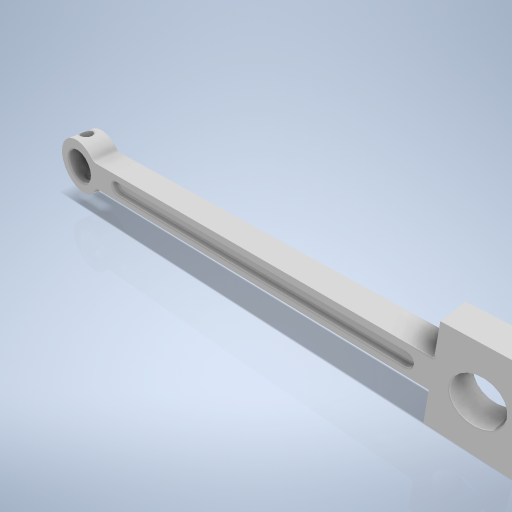
# Autodesk Inventor part: pleuel_rad_2
Saved by Autodesk Inventor 2024.2 (Build 282272000, 272)
## iProperties
Created: 2024-05-05
Part Number: pleuel_rad_2
Material: Generisch
Document SubType Name: Modeling
Designer: Fabri
Density: 1 g/cm^3
Appearance: Vorgabe
Author: Fabri
Autodesk Inventor part; units mm, degrees
ref_plane "YZ Plane" through (0, 0, 0) normal (1, 0, 0) x (0, 1, 0)
sketch "Skizze1" plane through (0, 0, 0) normal (0, 1, 0) x (-1, 0, 0)
  line L0 (0, 19.5) -> (-30, 19.5)
  line L1 (-30, 19.5) -> (-30, -19.5)
  line L2 (-30, -19.5) -> (0, -19.5)
  line L3 (0, -19.5) -> (0, 19.5)
  line L4 (0, 6) -> (169.4, 6)
  line L5 (169.4, 6) -> (169.4, -6)
  line L6 (169.4, -6) -> (0, -6)
  line L7 (0, -6) -> (0, 6)
  line L8 (0, 0) -> (-64.3399, 0) construction
  line L9 (9, 0) -> (145, 0) construction
  line L10 (9, 3) -> (145, 3)
  line L11 (145, -3) -> (9, -3)
  arc A0 (9, 3) -> (9, -3) centre (9, 0) ccw
  arc A1 (145, -3) -> (145, 3) centre (145, 0) ccw
  point P0 (169.4, 0)
  point P1 (-15, -19.5)
  point P2 (77, 0)
  point P3 (6, 0)
  point P4 (148, 0)
  dimension "d0" = 39
  dimension "d1" = 30
  dimension "d2" = 184.4
  dimension "d3" = 12
  dimension "d4" = 6
  dimension "d5" = 6
  dimension "d6" = 3
  dimension "d27" = 142
  constraints: 26 end point, 6 parallel, 6 point on circle, 4 midpoint, 4 tangent, 3 horizontal, 2 centre point, 2 perpendicular, 1 point on line, 1 symmetric about line, 2 other
  measures "d0" distance between parallel lines of L2 L0
  measures "d1" distance between parallel lines of L1 L3
  measures "d2" horizontal distance of point (-15, -19.5) point (169.4, 0)
  measures "d3" distance between parallel lines of L6 L4
  measures "d4" distance between parallel lines of L11 L10
  measures "d5" distance from line of L7 point (6, 0)
  measures "d6" distance between parallel lines of L6 L11
  measures "d27" distance of point (148, 0) point (6, 0)
extrude "Extrusion1" add sketch "Skizze1" along normal mid plane 12
extrude "Extrusion2" add sketch "Skizze1" along normal blind 3 contours L10 A1 L11 A0
extrude "Extrusion3" add sketch "Skizze1" against normal blind 3 contours L10 A1 L11 A0
sketch "Skizze2" plane through (0, 6, 0) normal (0, 1, 0) x (1, 0, 0)
  line L0 (30, 19.5) -> (0, 19.5) projected
  point P0 (0, 0)
  point P1 (15, 0)
  point P2 (15, 19.5)
  constraints: 1 horizontal alignment, 1 midpoint, 1 vertical alignment
hole "Bohrung1" at (15, 6, 0) direction (0, -1, 0) diameter 18 depth 12
ref_plane "Arbeitsebene1" through (0, 0, 0) normal (0, 1, 0) x (-1, 0, 0)
sketch "Skizze4" plane through (0, 0, 0) normal (0, 1, 0) x (-1, 0, 0)
  line L0 (169.4, 6) -> (169.4, -6) projected
  circle A0 centre (169.4, 0) radius 12
  point P0 (0, 0)
  dimension "d24" = 24
  constraints: 1 centre point, 1 midpoint
  measures "d24" diameter of A0
extrude "Extrusion4" add sketch "Skizze4" along normal mid plane 12
sketch "Skizze5" plane through (0, 0, 0) normal (0, 1, 0) x (-1, 0, 0)
  circle A0 centre (169.4, 0) radius 7.5
  arc A1 (159.0077, -6) -> (159.0077, 6) centre (169.4, 0) ccw projected
  point P0 (0, 0)
  dimension "d28" = 15
  constraints: 1 centre point, 1 coincident
  measures "d28" diameter of A0
extrude "Extrusion5" cut sketch "Skizze5" along normal mid plane 12
fillet "Rundung1" radius 3 2 edges at (-159.0077, 0, 6) (-159.0077, 0, -6)
ref_plane "Arbeitsebene2" through (0, 0, 12) normal (0, 0, 1) x (1, 0, 0)
sketch "Skizze6" plane through (0, 0, 12) normal (0, 0, 1) x (1, 0, 0)
  line L0 (-181.4, -6) -> (-181.4, 6) projected
  line L1 (-159.8, -6) -> (-159.8, 6) projected
  line L2 (-159.8, -6) -> (-159.8, -6) projected
  line L3 (-159.8, 6) -> (-159.8, -6) projected
  line L4 (-159.8, 6) -> (-159.8, 6) projected
  line L5 (-159.8, 6) -> (-181.4, 6) projected
  point P0 (0, 0)
  point P1 (-170.6, 0)
  point P2 (-181.4, 0)
  point P3 (-170.6, 6)
  constraints: 2 midpoint, 1 horizontal alignment, 1 vertical alignment
hole "Bohrung2" at (-170.6, 0, 12) direction (0, 0, -1) diameter 6 end through all
sketch "Skizze7" plane through (0, -6, 19.5) normal (-1, 0, 0) x (0, 0, 1)
  line L0 (-12, 0) -> (-27, 0) projected
  line L1 (-25.5, 0) -> (-39, 0) projected
  line L2 (-39, 0) -> (0, 0) projected
  line L3 (0, 0) -> (-13.5, 0) projected
  line L4 (-12.3, 0) -> (-13.5, 0) projected
  line L5 (-12.3, 0) -> (-26.7, 0) projected
  line L6 (-25.5, 0) -> (-26.7, 0) projected
  line L7 (-22.5, 0) -> (-16.5, 0) projected
  line L8 (-16.5, 0) -> (-22.5, 0) projected
  line L9 (-10.5, 0) -> (-28.5, 0) projected
  point P0 (-19.5, 6)
  point P1 (-6, 6)
  point P2 (-33, 6)
  point P3 (-6.75, 0)
  dimension "d48" = 6
  dimension "d50" = 13.5
  dimension "d51" = 13.5
  constraints: 2 horizontal alignment, 1 midpoint
  measures "d48" vertical distance of point (-6, 6) point (-6.75, 0)
  measures "d50" distance of point (-33, 6) point (-19.5, 6)
  measures "d51" distance of point (-19.5, 6) point (-6, 6)
hole "Bohrung3" at (0, 0, 13.5) at (0, 0, -13.5) direction (1, 0, 0) diameter 6 end through all
equation "\"d51\" = d50"
